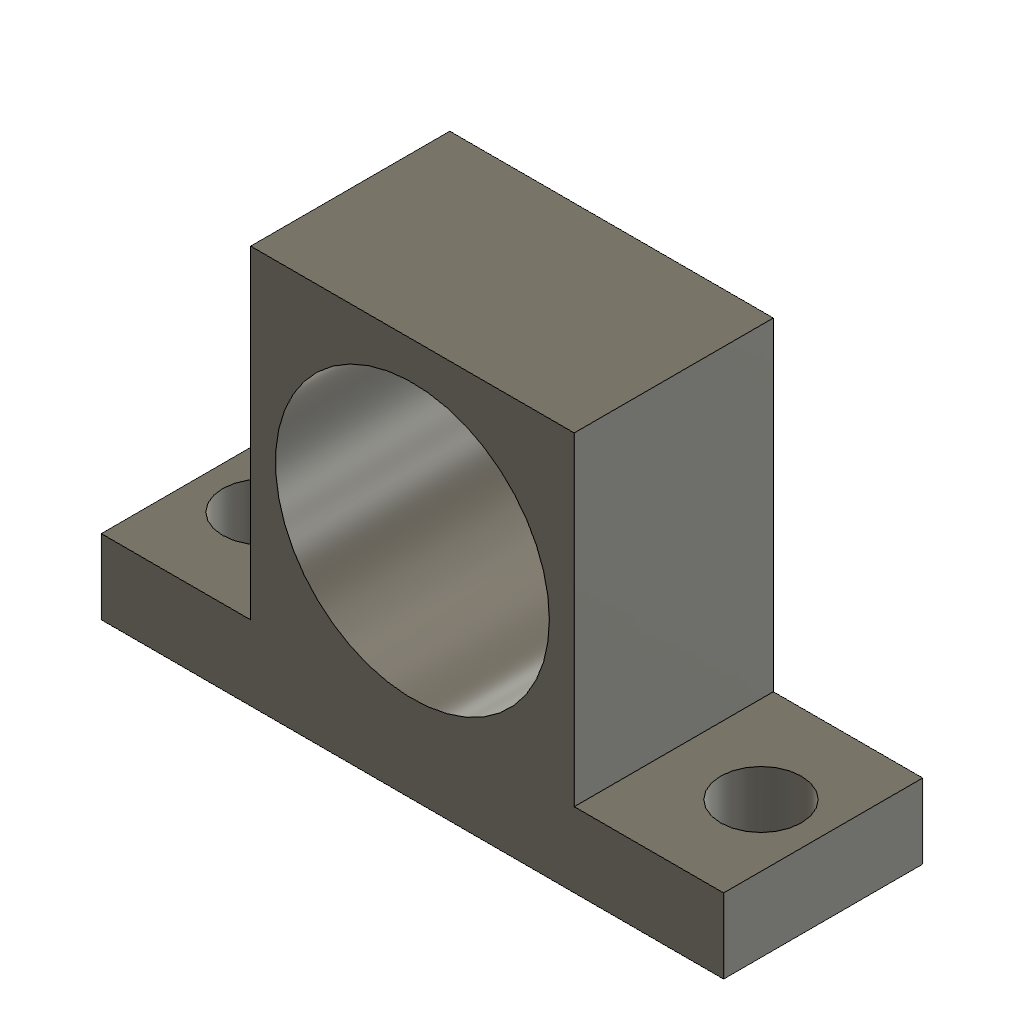
TankBot Wire Management (Autodesk Fusion 360 design; units mm, degrees)
Autodesk Fusion 360 part; units mm, degrees
box "BoxPrimitive1" add length 6 width 20 height 8 placed x (0, 0, 1) y (1, 0, 0) z (0, 1, 0) at (0, 0, 0)
box "BoxPrimitive2" cut length 5 width 6 height -6 placed x (0, 1, 0) y (0, 0, 1) z (1, 0, 0) at (20, 3, 0)
extrude "Extrude1" add 1 faces at (0, 2.6667, 4) along direction (-1, 0, 0) blind 5
box "BoxPrimitive3" cut length 5 width 6 height -6 placed x (0, 1, 0) y (0, 0, -1) z (-1, 0, 0) at (-5, 3, 6)
box "BoxPrimitive4" add length 2 width 3 height 1 placed x (0, -1, 0) y (1, 0, 0) z (0, 0, 1) at (3, 5, 6)
box "BoxPrimitive5" add length 2 width 3 height 1 placed x (0, -1, 0) y (1, 0, 0) z (0, 0, 1) at (9, 5, 6)
extrude "Extrude2" cut 1 faces at (5, 4.3333, 7) along direction (0, 0, -1) blind 7
extrude "Extrude3" cut 1 faces at (11, 4.3333, 7) along direction (0, 0, -1) blind 7
hole "Hole3" at (-2.5, 3, 3) direction (0, -1, 0) diameter 3.25 depth 3 tip angle 180
hole "Hole4" at (17.5, 3, 3) direction (0, -1, 0) diameter 3.25 depth 3 tip angle 180
extrude "Extrude4" add 1 faces at (9.6667, 8, 2) along direction (0, 1, 0) blind 3
extrude "Extrude5" add 1 faces at (7, 9, 6) along direction (0, 0, 1) blind 1
extrude "Extrude6" add 1 faces at (7, 9, 0) along direction (0, 0, -1) blind 1
extrude "Extrude7" add 1 faces at (9.6667, 11, 1.6667) along direction (0, 1, 0) blind 2
extrude "Extrude8" cut 1 faces at (10, 5, 4.3333) along direction (0, 1, 0) blind 1
extrude "Extrude9" cut 1 faces at (5, 5, 1.6667) along direction (0, 1, 0) blind 1
delete_face "DeleteFace1" 1 faces at (4, 3, 1.6667)
delete_face "DeleteFace2" 1 faces at (11, 3, 1.6667)
extrude "Extrude10" add 1 faces at (5.3333, 13, 4.3333) along direction (0, 1, 0) blind 3
hole "Hole10" at (7.5, 9, 7) direction (0, 0, -1) diameter 11 depth 160 tip angle 180
